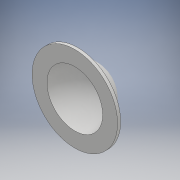
# Autodesk Inventor part: Dome
Saved by Autodesk Inventor 2017 (Build 210142000, 142)
## iProperties
Created: 2018-02-08
Part Number: Dome
Material: Generic
Document SubType Name: Modeling
Designer: Arjuna
Density: 1 g/cm^3
Appearance: Default
Author: Arjuna
Autodesk Inventor part; units mm, degrees
ref_plane "YZ Plane" through (0, 0, 0) normal (1, 0, 0) x (0, 1, 0)
ref_plane "XZ Plane" through (0, 0, 0) normal (0, 1, 0) x (-1, 0, 0)
ref_plane "XY Plane" through (0, 0, 0) normal (0, 0, 1) x (1, 0, 0)
sketch "Sketch1" plane through (0, 0, 0) normal (0, 0, 1) x (1, 0, 0)
  line L0 (22.5, 0) -> (22.5, 0)
  line L1 (22.5, 0) -> (34.5, 0)
  line L2 (34.5, 0) -> (34.5, 2.5)
  line L3 (34.5, 2.5) -> (24.3721, 2.5)
  line L4 (0, 24.5) -> (0, 22.5)
  arc A0 (22.5, 0) -> (0, 22.5) centre (0, 0) ccw
  arc A1 (24.5, 0) -> (0, 24.5) centre (0, 0) ccw
  line L5 (0, -5.9148) -> (0, 35.4889) projected
  point P0 (0, 0)
  dimension "d11" = 22.5
  dimension "d12" = 22.5
  dimension "d13" = 24.5
  dimension "d14" = 2
  dimension "d15" = 2.5
  dimension "d16" = 0
  dimension "d17" = 2
  dimension "d18" = 12
  constraints: 10 end point, 5 point on circle, 2 centre point, 2 perpendicular, 1 point on line
  measures "d11" distance between parallel lines of L5 L0
  measures "d12" radius of A0
  measures "d13" radius of A1
  measures "d14" distance of L4.start L4.end
  measures "d15" distance between parallel lines of L1 L3
  measures "d16" distance of L0.start L0.end
  measures "d17" distance of A1.start L0.start
  measures "d18" distance of L0.end L1.end
revolve "Revolution1" add sketch "Sketch1" angle 360 about axis through (0, -10, 0) along (0, 1, 0)
equation "\"d12\" = d11"
equation "\"d13\" = d12 + d17"
equation "\"d14\" = d17"
body "Solid1"
